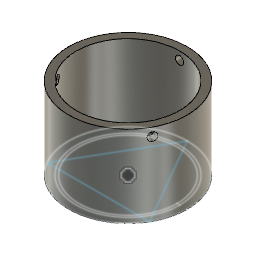
Eschenbach 33213 Barlow Lens Adapter (Autodesk Fusion 360 design; units mm, degrees)
part number: 2026-06-22-15-08-21-655
Autodesk Fusion 360 part; units mm, degrees
sketch "Adapter Sketch" plane through (0, 0, 0) normal (0, 0, 1) x (1, 0, 0)
  circle A0 centre (0, 0) radius 25.25
  circle A1 centre (0, 0) radius 29
  circle A2 centre (0, 0) radius 24
  line L0 (25.0221, -14.4721) -> (0.0222, 28.9059)
  line L1 (0.0222, 28.9059) -> (-25.0443, -14.4337)
  line L2 (-25.0443, -14.4337) -> (25.0221, -14.4721)
  dimension "d1" = 50.5
  dimension "d2" = 58
  dimension "d3" = 48
  constraint coincident A0.centre A1.centre
  constraint concentric A0 A1
  measures "d1" diameter of A0
  measures "d2" diameter of A1
  measures "d3" diameter of A2
extrude "Extrude1" add sketch "Adapter Sketch" along normal blind 1 contours A0 A2 L0 | A0 A2 L0 L1 | A0 A2 L0 L2 | A0 A2 L1 | A0 A2 L2 | A0 A2 L1 L2
extrude "Extrude2" add sketch "Adapter Sketch" along normal blind 40 contours A0 L0 L1 | A0 L0 L2 | A0 L1 L2 | A1
hole "Hole1" at (25.6055, -13.6147, 35.9754) direction (-0.882948, 0.469472, 0) diameter 4 depth 5 tip angle 180
hole "Hole2" at (-25.1147, -14.5, 35.7941) direction (0.866025, 0.5, 0) diameter 4 depth 5 tip angle 180
hole "Hole3" at (0, 29, 36.074) direction (0, -1, 0) diameter 4 depth 5 tip angle 180
named bodies: "Adapter"
